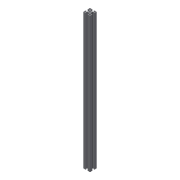
# Autodesk Inventor part: Propile_202040
Saved by Autodesk Inventor 2019 (Build 230136000, 136)
## iProperties
Created: 2019-05-03
Part Number: Propile_202040
Material: 일반
Document SubType Name: Modeling
Designer: hinmo
Density: 1 g/cm^3
Appearance: 기본값
Author: hinmo
Autodesk Inventor part; units mm, degrees
ref_plane "YZ Plane" through (0, 0, 0) normal (1, 0, 0) x (0, 1, 0)
ref_plane "XZ Plane" through (0, 0, 0) normal (0, 1, 0) x (-1, 0, 0)
ref_plane "XY Plane" through (0, 0, 0) normal (0, 0, 1) x (1, 0, 0)
sketch "스케치1" plane through (0, 0, 0) normal (0, 1, 0) x (-1, 0, 0)
  circle A0 centre (492.8246, -160.4273) radius 2.15 projected
  circle A1 centre (499.8246, -167.4273) radius 2 projected
  circle A2 centre (499.8246, -153.4273) radius 2 projected
  circle A3 centre (485.8246, -153.4273) radius 2 projected
  circle A4 centre (485.8246, -167.4273) radius 2 projected
  arc A5 (490.1746, -150.7273) -> (489.8746, -150.4273) centre (489.8746, -150.7273) ccw projected
  line L0 (489.8746, -150.4273) -> (483.1246, -150.4273) projected
  arc A6 (483.1246, -150.4273) -> (482.8246, -150.7273) centre (483.1246, -150.7273) ccw projected
  line L1 (482.8246, -150.7273) -> (482.8246, -157.4773) projected
  arc A7 (482.8246, -157.4773) -> (483.1246, -157.7773) centre (483.1246, -157.4773) ccw projected
  line L2 (483.1246, -157.7773) -> (484.3246, -157.7773) projected
  line L3 (484.3246, -157.7773) -> (484.3246, -156.2773) projected
  line L4 (484.3246, -156.2773) -> (487.8246, -156.2773) projected
  arc A8 (487.8246, -164.5773) -> (487.8246, -156.2773) centre (482.5646, -160.4273) ccw projected
  line L5 (487.8246, -164.5773) -> (484.3246, -164.5773) projected
  line L6 (484.3246, -164.5773) -> (484.3246, -163.0773) projected
  line L7 (484.3246, -163.0773) -> (483.1246, -163.0773) projected
  arc A9 (483.1246, -163.0773) -> (482.8246, -163.3773) centre (483.1246, -163.3773) ccw projected
  line L8 (482.8246, -163.3773) -> (482.8246, -170.1273) projected
  arc A10 (482.8246, -170.1273) -> (483.1246, -170.4273) centre (483.1246, -170.1273) ccw projected
  line L9 (483.1246, -170.4273) -> (489.8746, -170.4273) projected
  arc A11 (489.8746, -170.4273) -> (490.1746, -170.1273) centre (489.8746, -170.1273) ccw projected
  line L10 (490.1746, -170.1273) -> (490.1746, -168.9273) projected
  line L11 (490.1746, -168.9273) -> (488.6746, -168.9273) projected
  line L12 (488.6746, -168.9273) -> (488.6746, -165.4273) projected
  arc A12 (496.9746, -165.4273) -> (488.6746, -165.4273) centre (492.8246, -170.6873) ccw projected
  line L13 (496.9746, -165.4273) -> (496.9746, -168.9273) projected
  line L14 (496.9746, -168.9273) -> (495.4746, -168.9273) projected
  line L15 (495.4746, -168.9273) -> (495.4746, -170.1273) projected
  arc A13 (495.4746, -170.1273) -> (495.7746, -170.4273) centre (495.7746, -170.1273) ccw projected
  line L16 (495.7746, -170.4273) -> (502.5246, -170.4273) projected
  arc A14 (502.5246, -170.4273) -> (502.8246, -170.1273) centre (502.5246, -170.1273) ccw projected
  line L17 (502.8246, -170.1273) -> (502.8246, -163.3773) projected
  arc A15 (502.8246, -163.3773) -> (502.5246, -163.0773) centre (502.5246, -163.3773) ccw projected
  line L18 (502.5246, -163.0773) -> (501.3246, -163.0773) projected
  line L19 (501.3246, -163.0773) -> (501.3246, -164.5773) projected
  line L20 (501.3246, -164.5773) -> (497.8246, -164.5773) projected
  arc A16 (497.8246, -156.2773) -> (497.8246, -164.5773) centre (503.0846, -160.4273) ccw projected
  line L21 (497.8246, -156.2773) -> (501.3246, -156.2773) projected
  line L22 (501.3246, -156.2773) -> (501.3246, -157.7773) projected
  line L23 (501.3246, -157.7773) -> (502.5246, -157.7773) projected
  arc A17 (502.5246, -157.7773) -> (502.8246, -157.4773) centre (502.5246, -157.4773) ccw projected
  line L24 (502.8246, -157.4773) -> (502.8246, -150.7273) projected
  arc A18 (502.8246, -150.7273) -> (502.5246, -150.4273) centre (502.5246, -150.7273) ccw projected
  line L25 (502.5246, -150.4273) -> (495.7746, -150.4273) projected
  arc A19 (495.7746, -150.4273) -> (495.4746, -150.7273) centre (495.7746, -150.7273) ccw projected
  line L26 (495.4746, -150.7273) -> (495.4746, -151.9273) projected
  line L27 (495.4746, -151.9273) -> (496.9746, -151.9273) projected
  line L28 (496.9746, -151.9273) -> (496.9746, -155.4273) projected
  arc A20 (488.6746, -155.4273) -> (496.9746, -155.4273) centre (492.8246, -150.1673) ccw projected
  line L29 (488.6746, -155.4273) -> (488.6746, -151.9273) projected
  line L30 (488.6746, -151.9273) -> (490.1746, -151.9273) projected
  line L31 (490.1746, -151.9273) -> (490.1746, -150.7273) projected
  circle A21 centre (0, 0) radius 2.15
  circle A22 centre (7, -7) radius 2
  circle A23 centre (7, 7) radius 2
  circle A24 centre (-7, 7) radius 2
  circle A25 centre (-7, -7) radius 2
  arc A26 (-2.65, 9.7) -> (-2.95, 10) centre (-2.95, 9.7) ccw
  line L32 (-2.95, 10) -> (-9.7, 10)
  arc A27 (-9.7, 10) -> (-10, 9.7) centre (-9.7, 9.7) ccw
  line L33 (-10, 9.7) -> (-10, 2.95)
  arc A28 (-10, 2.95) -> (-9.7, 2.65) centre (-9.7, 2.95) ccw
  line L34 (-9.7, 2.65) -> (-8.5, 2.65)
  line L35 (-8.5, 2.65) -> (-8.5, 4.15)
  line L36 (-8.5, 4.15) -> (-5, 4.15)
  arc A29 (-5, -4.15) -> (-5, 4.15) centre (-10.26, 0) ccw
  line L37 (-5, -4.15) -> (-8.5, -4.15)
  line L38 (-8.5, -4.15) -> (-8.5, -2.65)
  line L39 (-8.5, -2.65) -> (-9.7, -2.65)
  arc A30 (-9.7, -2.65) -> (-10, -2.95) centre (-9.7, -2.95) ccw
  line L40 (-10, -2.95) -> (-10, -9.7)
  arc A31 (-10, -9.7) -> (-9.7, -10) centre (-9.7, -9.7) ccw
  line L41 (-9.7, -10) -> (-2.95, -10)
  arc A32 (-2.95, -10) -> (-2.65, -9.7) centre (-2.95, -9.7) ccw
  line L42 (-2.65, -9.7) -> (-2.65, -8.5)
  line L43 (-2.65, -8.5) -> (-4.15, -8.5)
  line L44 (-4.15, -8.5) -> (-4.15, -5)
  arc A33 (4.15, -5) -> (-4.15, -5) centre (0, -10.26) ccw
  line L45 (4.15, -5) -> (4.15, -8.5)
  line L46 (4.15, -8.5) -> (2.65, -8.5)
  line L47 (2.65, -8.5) -> (2.65, -9.7)
  arc A34 (2.65, -9.7) -> (2.95, -10) centre (2.95, -9.7) ccw
  line L48 (2.95, -10) -> (9.7, -10)
  arc A35 (9.7, -10) -> (10, -9.7) centre (9.7, -9.7) ccw
  line L49 (10, -9.7) -> (10, -2.95)
  arc A36 (10, -2.95) -> (9.7, -2.65) centre (9.7, -2.95) ccw
  line L50 (9.7, -2.65) -> (8.5, -2.65)
  line L51 (8.5, -2.65) -> (8.5, -4.15)
  line L52 (8.5, -4.15) -> (5, -4.15)
  arc A37 (5, 4.15) -> (5, -4.15) centre (10.26, 0) ccw
  line L53 (5, 4.15) -> (8.5, 4.15)
  line L54 (8.5, 4.15) -> (8.5, 2.65)
  line L55 (8.5, 2.65) -> (9.7, 2.65)
  arc A38 (9.7, 2.65) -> (10, 2.95) centre (9.7, 2.95) ccw
  line L56 (10, 2.95) -> (10, 9.7)
  arc A39 (10, 9.7) -> (9.7, 10) centre (9.7, 9.7) ccw
  line L57 (9.7, 10) -> (2.95, 10)
  arc A40 (2.95, 10) -> (2.65, 9.7) centre (2.95, 9.7) ccw
  line L58 (2.65, 9.7) -> (2.65, 8.5)
  line L59 (2.65, 8.5) -> (4.15, 8.5)
  line L60 (4.15, 8.5) -> (4.15, 5)
  arc A41 (-4.15, 5) -> (4.15, 5) centre (0, 10.26) ccw
  line L61 (-4.15, 5) -> (-4.15, 8.5)
  line L62 (-4.15, 8.5) -> (-2.65, 8.5)
  line L63 (-2.65, 8.5) -> (-2.65, 9.7)
  point P0 (0, 0)
  constraints: 64 end point, 32 point on circle, 21 centre point
extrude "돌출1" add sketch "스케치1" along normal blind 400 contours L63 L62 L61 A41 L60 L59 L58 A40 L57 A39 L56 A38 L55 L54 L53 A37 L52 L51 L50 A36 L49 A35 L48 A34 L47 L46 L45 A33 L44 L43 L42 A32 L41 A31 L40 A30 L39 L38 L37 A29 L36 L35 L34 A28 L33 A27 L32 A26
